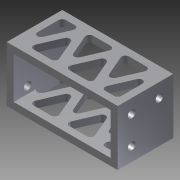
# Autodesk Inventor part: 1x2 Aluminum Tube Corner Post
Saved by Autodesk Inventor 2012 (Build 160160000, 160)
## iProperties
Created: 2012-12-19
Part Number: 1x2 Aluminum Tube Corner Post
Material: Default
Document SubType Name: Modeling
Designer: Administrator
Density: 1 g/cm^3
Author: Administrator
Autodesk Inventor part; units mm, degrees
ref_plane "YZ Plane" through (0, 0, 0) normal (1, 0, 0) x (0, 1, 0)
ref_plane "XZ Plane" through (0, 0, 0) normal (0, 1, 0) x (-1, 0, 0)
ref_plane "XY Plane" through (0, 0, 0) normal (0, 0, 1) x (1, 0, 0)
sketch "Sketch1" plane through (0, 0, 0) normal (0, 0, 1) x (1, 0, 0)
  line L0 (0, 0) -> (50.8, 0)
  line L1 (50.8, 0) -> (50.8, 25.4)
  line L2 (50.8, 25.4) -> (0, 25.4)
  line L3 (0, 25.4) -> (0, 0)
  line L4 (3.175, 22.225) -> (47.625, 22.225)
  line L5 (47.625, 22.225) -> (47.625, 3.175)
  line L6 (47.625, 3.175) -> (3.175, 3.175)
  line L7 (3.175, 3.175) -> (3.175, 22.225)
  dimension "d0" = 50.8
  dimension "d1" = 25.4
  dimension "d2" = 3.175
  dimension "d3" = 3.175
  dimension "d4" = 3.175
  dimension "d5" = 3.175
  constraints: 16 end point, 4 parallel, 2 horizontal, 2 perpendicular
  measures "d0" distance of L0.start L0.end
  measures "d1" distance of L2.end L0.start
  measures "d2" distance between parallel lines of L2 L4
  measures "d3" distance between parallel lines of L3 L7
  measures "d4" distance between parallel lines of L6 L0
  measures "d5" distance between parallel lines of L5 L1
extrude "Extrusion1" add sketch "Sketch1" along normal blind 25.4
sketch "Sketch2" plane through (0, 25.4, 0) normal (0, 1, 0) x (1, 0, 0)
  line L0 (0, -25.4) -> (50.8, -25.4) projected
  line L1 (50.8, 0) -> (50.8, -25.4) projected
  line L2 (0, 0) -> (0, -25.4) projected
  line L3 (3.175, -22.225) -> (3.175, -3.175)
  line L4 (47.625, -22.225) -> (3.175, -22.225)
  line L5 (3.175, -3.175) -> (47.625, -3.175)
  line L6 (27.7711, -3.175) -> (21.3007, -18.2093)
  line L7 (29.4993, -3.175) -> (21.3007, -22.225) construction
  line L8 (29.4993, -7.1907) -> (23.0289, -22.225)
  line L9 (35.9698, -22.225) -> (29.4993, -7.1907)
  line L10 (37.698, -22.225) -> (29.4993, -3.175) construction
  line L11 (37.698, -18.2093) -> (31.2276, -3.175)
  line L12 (44.1684, -3.175) -> (37.698, -18.2093)
  line L13 (45.8967, -3.175) -> (37.698, -22.225) construction
  line L14 (39.4263, -22.225) -> (47.625, -3.175)
  line L15 (47.625, -3.175) -> (47.625, -22.225)
  line L16 (21.3007, -18.2093) -> (14.8302, -3.175)
  line L17 (21.3007, -22.225) -> (13.102, -3.175) construction
  line L18 (19.5724, -22.225) -> (13.102, -7.1907)
  line L19 (13.102, -7.1907) -> (6.6316, -22.225)
  line L20 (13.102, -3.175) -> (4.9033, -22.225) construction
  line L21 (3.175, -22.225) -> (11.3737, -3.175)
  line L22 (50.8, 0) -> (0, 0) projected
  dimension "d9" = 1.5875
  dimension "d10" = 3.175
  dimension "d11" = 1.5875
  dimension "d12" = 3.175
  dimension "d13" = 1.5875
  dimension "d14" = 3.175
  dimension "d15" = 1.5875
  dimension "d16" = 3.175
  dimension "d17" = 1.5875
  dimension "d18" = 3.175
  dimension "d19" = 23.286
  dimension "d20" = 46.572
  dimension "d21" = 46.572
  dimension "d22" = 46.572
  dimension "d23" = 46.572
  dimension "d24" = 3.175
  dimension "d26" = 3.175
  dimension "d27" = 3.175
  dimension "d32" = 3.175
  constraints: 34 end point, 6 parallel, 1 point on line, 1 vertical, 23 other
  measures "d9" distance between parallel lines of L13 L14
  measures "d10" distance between parallel lines of L12 L14
  measures "d11" distance between parallel lines of L10 L11
  measures "d12" distance between parallel lines of L9 L11
  measures "d13" distance between parallel lines of L8 L7
  measures "d14" distance between parallel lines of L8 L6
  measures "d15" distance between parallel lines of L17 L16
  measures "d16" distance between parallel lines of L16 L18
  measures "d17" distance between parallel lines of L20 L19
  measures "d18" distance between parallel lines of L19 L21
  measures "d19" angle of L15 L14
  measures "d20" angle of L12 L11
  measures "d21" angle of L9 L8
  measures "d22" angle of L6 L16
  measures "d23" angle of L18 L19
  measures "d24" distance between parallel lines of L2 L3
  measures "d27" distance between parallel lines of L1 L15
extrude "Extrusion2" cut sketch "Sketch2" against normal blind 76.2 contours L3 L5 L21 | L19 L18 L4 | L5 L6 L16 | L8 L9 L4 | L5 L12 L11 | L14 L15 L4
fillet "Fillet1" radius 1.5875 18 edges at (3.175, 23.8125, 3.175) (11.3737, 23.8125, 3.175) (3.175, 23.8125, 22.225) (13.102, 23.8125, 7.1907) (6.6316, 23.8125, 22.225) (19.5724, 23.8125, 22.225) (14.8302, 23.8125, 3.175) (21.3007, 23.8125, 18.2093) (27.7711, 23.8125, 3.175) (29.4993, 23.8125, 7.1907) (23.0289, 23.8125, 22.225) (35.9698, 23.8125, 22.225) (31.2276, 23.8125, 3.175) (37.698, 23.8125, 18.2093) (44.1684, 23.8125, 3.175) (47.625, 23.8125, 3.175) (39.4263, 23.8125, 22.225) (47.625, 23.8125, 22.225)
fillet "Fillet2" radius 1.5875 18 edges at (11.3737, 1.5875, 3.175) (3.175, 1.5875, 3.175) (3.175, 1.5875, 22.225) (6.6316, 1.5875, 22.225) (13.102, 1.5875, 7.1907) (19.5724, 1.5875, 22.225) (21.3007, 1.5875, 18.2093) (14.8302, 1.5875, 3.175) (27.7711, 1.5875, 3.175) (29.4993, 1.5875, 7.1907) (23.0289, 1.5875, 22.225) (35.9698, 1.5875, 22.225) (37.698, 1.5875, 18.2093) (31.2276, 1.5875, 3.175) (44.1684, 1.5875, 3.175) (47.625, 1.5875, 3.175) (39.4263, 1.5875, 22.225) (47.625, 1.5875, 22.225)
sketch "Sketch3" plane through (50.8, 0, 0) normal (1, 0, 0) x (0, 0, -1)
  line L0 (-25.4, 25.4) -> (-25.4, 0) projected
  line L1 (0, 0) -> (-25.4, 0) projected
  line L2 (0, 0) -> (0, 25.4) projected
  line L3 (0, 25.4) -> (-25.4, 25.4) projected
  circle A0 centre (-19.05, 19.05) radius 1.7272
  circle A1 centre (-19.05, 6.35) radius 1.7272
  circle A2 centre (-6.35, 19.05) radius 1.7272
  dimension "d33" = 3.4544
  dimension "d34" = 6.35
  dimension "d35" = 6.35
  dimension "d36" = 6.35
  dimension "d37" = 6.35
  constraints: 3 centre point, 2 equal radius, 1 horizontal alignment, 1 vertical alignment
  measures "d33" diameter of A0
  measures "d34" distance from line of L3 A0.centre
  measures "d35" distance from line of L0 A0.centre
  measures "d36" distance from line of L2 A2.centre
  measures "d37" distance from line of L1 A1.centre
extrude "Extrusion3" cut sketch "Sketch3" against normal through all contours A0 | A1 | A2
equation "\"d3\" = d2"
equation "\"d4\" = d2"
equation "\"d5\" = d2"
equation "\"d10\" = 2 * d9"
equation "\"d11\" = d9"
equation "\"d12\" = d10"
equation "\"d13\" = d11"
equation "\"d15\" = d13"
equation "\"d16\" = d14"
equation "\"d17\" = d15"
equation "\"d18\" = d16"
equation "\"d20\" = 2 * d19"
equation "\"d21\" = d20"
equation "\"d22\" = d21"
equation "\"d23\" = d22"
equation "\"d36\" = d35"
equation "\"d37\" = d34"
body "Solid1"
